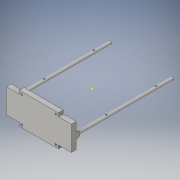
# Autodesk Inventor part: Linear Actuator Piece 1
Saved by Autodesk Inventor 2016 (Build 200138000, 138)
## iProperties
Created: 2015-12-05
Part Number: Linear Actuator Piece 1
Material: Generic
Document SubType Name: Modeling
Designer: Javier
Density: 1 g/cm^3
Appearance: Default
Author: Javier
Autodesk Inventor part; units mm, degrees
ref_plane "YZ Plane" through (0, 0, 0) normal (1, 0, 0) x (0, 1, 0)
sketch "Sketch1" plane through (0, 0, 0) normal (0, 0, 1) x (1, 0, 0)
  line L0 (-127, 0) -> (0, 0)
  line L1 (0, 0) -> (139.7, 0)
  circle A0 centre (-127, 0) radius 6.35
  dimension "d0" = 127
  dimension "d1" = 139.7
  constraints: 4 end point, 1 centre point, 1 coincident, 1 horizontal, 1 point on line
  measures "d0" distance of L0.start L0.end
  measures "d1" distance of L0.end L1.end
extrude "Extrusion1" add sketch "Sketch1" along normal blind 203.2
sketch "Sketch2" plane through (0, 0, 0) normal (0, 0, 1) x (1, 0, 0)
  circle A0 centre (-127, 0) radius 6.35 projected
  line L0 (-127, 0) -> (0, 0)
  line L1 (0, 0) -> (127, 0)
  circle A1 centre (127, 0) radius 6.35
  dimension "d4" = 127
  dimension "d5" = 12.7
  constraints: 4 end point, 1 centre point, 1 coincident, 1 horizontal, 1 point on line
  measures "d4" distance of L0.end L1.end
  measures "d5" diameter of A1
extrude "Extrusion2" add sketch "Sketch2" along normal blind 203.2 contours A1
sketch "Sketch3" plane through (0, 0, 0) normal (1, 0, 0) x (0, 1, 0)
  circle A0 centre (0, 196.3216) radius 12.7
  point P0 (0, 0)
  dimension "d17" = 25.4
  constraints: 1 centre point, 1 other
  measures "d17" diameter of A0
extrude "Extrusion3" add sketch "Sketch3" along normal mid plane 266.7
ref_plane "Work Plane1" through (0, 0, 203.2) normal (0, 0, 1) x (1, 0, 0)
ref_plane "Work Plane2" through (0, 0, 212.344) normal (0, 0, 1) x (1, 0, 0)
sketch "Sketch8" plane through (0, 0, 0) normal (0, 1, 0) x (-1, 0, 0)
  point P0 (0, 0)
sketch "Sketch9" plane through (0, 0, 0) normal (0, 1, 0) x (-1, 0, 0)
  line L0 (80, 219.075) -> (80, 199.075)
  line L1 (80, 199.075) -> (-80, 199.075)
  line L2 (-80, 199.075) -> (-80, 219.075)
  line L3 (0, 231.775) -> (0, 174.625)
  line L4 (-80, 219.075) -> (0, 219.075)
  line L5 (80, 219.075) -> (0, 219.075)
  point P0 (0, 0)
  dimension "d29" = 20
  dimension "d69" = 80
  dimension "d70" = 80
  constraints: 12 end point, 3 perpendicular, 3 vertical, 1 collinear, 1 point on line
  measures "d29" distance of L0.start L0.end
  measures "d69" distance of L2.end L4.end
  measures "d70" distance of L0.start L4.end
extrude "Extrusion8" add sketch "Sketch9" along normal mid plane 128
sketch "Sketch10" plane through (0, 0, 0) normal (0, 0, 1) x (1, 0, 0)
  line L0 (-70, 54) -> (70, 54)
  circle A0 centre (-70, 54) radius 4
  circle A1 centre (70, 54) radius 4
  line L1 (-80, 64) -> (-80, 12.3979) projected
  line L2 (80, 64) -> (80, 12.3979) projected
  line L3 (-80, 64) -> (80, 64)
  point P0 (0, 0)
  dimension "d32" = 140
  dimension "d33" = 10
  dimension "d34" = 8
  dimension "d35" = 8
  dimension "d71" = 10
  dimension "d72" = 10
  constraints: 4 end point, 2 centre point, 2 coincident, 2 horizontal
  measures "d32" distance of L0.start L0.end
  measures "d33" distance from line of L3 L0.end
  measures "d34" diameter of A0
  measures "d35" diameter of A1
  measures "d71" distance from line of L1 L0.start
  measures "d72" distance from line of L2 L0.end
extrude "Extrusion9" cut sketch "Sketch10" along normal blind 240
sketch "Sketch11" plane through (0, 0, 212.344) normal (0, 0, 1) x (1, 0, 0)
  line L0 (-80, -64) -> (80, -64) projected
  line L1 (-80, -64) -> (80, -64)
  line L2 (0, -19.075) -> (0, -95.275)
  line L3 (-70, -54) -> (0, -54)
  line L4 (0, -54) -> (70, -54)
  circle A0 centre (-70, -54) radius 4
  circle A1 centre (70, -54) radius 4
  point P0 (0, 0)
  dimension "d48" = 70
  dimension "d49" = 70
  dimension "d50" = 10
  dimension "d51" = 8
  dimension "d52" = 8
  constraints: 8 end point, 2 centre point, 2 coincident, 2 point on line, 1 collinear, 1 perpendicular, 1 vertical
  measures "d48" distance of L3.start L3.end
  measures "d49" distance of L3.end L4.end
  measures "d50" distance between parallel lines of L0 L3
  measures "d51" diameter of A0
  measures "d52" diameter of A1
extrude "Extrusion10" cut sketch "Sketch11" along normal mid plane 30
sketch "Sketch12" plane through (0, 0, 0) normal (0, 1, 0) x (-1, 0, 0)
  line L0 (80, 199.075) -> (-80, 199.075) projected
  line L1 (80, 199.075) -> (133.35, 199.075)
  line L2 (133.35, 183.6216) -> (133.35, 209.0216) projected
  line L3 (80, 219.075) -> (-80, 219.075) projected
  line L4 (80, 219.075) -> (133.35, 219.075)
  line L5 (133.35, 219.075) -> (133.35, 199.075)
  line L6 (-80, 219.075) -> (-133.35, 219.075)
  line L7 (-133.35, 209.0216) -> (-133.35, 183.6216) projected
  line L8 (-133.35, 219.075) -> (-133.35, 199.075)
  line L9 (-80, 199.075) -> (-133.35, 199.075)
  point P0 (0, 0)
  constraints: 12 end point, 4 point on line, 2 collinear, 2 perpendicular, 1 horizontal
extrude "Extrusion11" add sketch "Sketch12" along normal mid plane 100
thread "Thread12" size "M8x1.25" class "6H" standard "ANSI Metric M Profile" full length
thread "Thread13" size "M8x1.25" class "6H" standard "ANSI Metric M Profile" full length
thread "Thread14" size "M8x1.25" class "6H" standard "ANSI Metric M Profile" full length
thread "Thread15" size "M8x1.25" class "6H" standard "ANSI Metric M Profile" full length
sketch "Sketch13" plane through (0, 0, 0) normal (0, 0, 1) x (1, 0, 0)
  circle A0 centre (-127, 0) radius 6.35
  line L0 (133.35, 0) -> (133.35, 12.7) projected
  circle A1 centre (127, 0) radius 6.35
  point P0 (0, 0)
  point P1 (133.35, 12.3979)
  constraints: 1 centre point, 1 horizontal alignment, 2 other
extrude "Extrusion12" add sketch "Sketch13" against normal blind 200
sketch "Sketch14" plane through (0, 0, 0) normal (0, 1, 0) x (-1, 0, 0)
  circle A0 centre (127, -149.225) radius 4.7625
  circle A1 centre (-127, -149.225) radius 4.7625
  line L0 (0, -204.7875) -> (0, 163.5125)
  line L1 (311.15, -31.4767) -> (-300.0375, -31.4767)
  line L2 (127, -212.725) -> (127, 163.5125)
  line L3 (120.65, -200) -> (120.65, 183.6216) projected
  line L4 (-127, -212.725) -> (-127, 174.625)
  line L5 (310.3631, -133.0767) -> (-296.0619, -133.0767)
  line L6 (311.15, 70.1233) -> (-300.0375, 70.1233)
  line L7 (103.1875, 183.6216) -> (306.3875, 183.6216)
  circle A2 centre (127, -133.0767) radius 3.175
  circle A3 centre (-127, -133.0767) radius 3.175
  circle A4 centre (127, 70.1233) radius 3.175
  circle A5 centre (-127, 70.1233) radius 3.175
  point P0 (0, 0)
  dimension "d84" = 101.6
  dimension "d85" = 203.2
  dimension "d86" = 254
  dimension "d87" = 113.4983
  dimension "d88" = 6.35
  dimension "d89" = 6.35
  dimension "d90" = 6.35
  dimension "d91" = 6.35
  constraints: 14 end point, 8 point on line, 6 centre point, 4 horizontal, 3 parallel, 2 vertical
  measures "d84" distance between parallel lines of L6 L1
  measures "d85" distance between parallel lines of L6 L5
  measures "d86" distance between parallel lines of L4 L2
  measures "d87" distance between parallel lines of L7 L6
  measures "d88" diameter of A2
  measures "d89" diameter of A3
  measures "d90" diameter of A4
  measures "d91" diameter of A5
extrude "Extrusion13" cut sketch "Sketch14" along normal mid plane 150 contours A2 L5 L2 | L2 L5 A2 | L5 A2 L2 | L2 A2 L5 | A4 L6 L2 | L2 L6 A4 | A3 L4 L5 | L5 L4 A3 | L6 A4 L2 | L2 A4 L6 | L5 A3 L4 | L4 A3 L5 | A5 L4 L6 | L6 L4 A5 | A5 L6 L4 | L6 A5 L4
thread "Thread16" size "M7x1" class "6H" standard "ANSI Metric M Profile" full length
thread "Thread17" size "M7x1" class "6H" standard "ANSI Metric M Profile" full length
thread "Thread18" size "M7x1" class "6H" standard "ANSI Metric M Profile" full length
thread "Thread19" size "M7x1" class "6H" standard "ANSI Metric M Profile" full length
body "Solid1"
